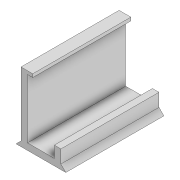
# Autodesk Inventor part: WagoHolder
Saved by Autodesk Inventor 2021 (Build 250183000, 183)
## iProperties
Created: 2021-07-30
Part Number: WagoHolder
Material: Generisch
Document SubType Name: Modeling
Designer: Rama
Density: 1 g/cm^3
Appearance: Vorgabe
Author: Rama
Autodesk Inventor part; units mm, degrees
ref_plane "YZ Plane" through (0, 0, 0) normal (1, 0, 0) x (0, 1, 0)
ref_plane "XZ Plane" through (0, 0, 0) normal (0, 1, 0) x (-1, 0, 0)
ref_plane "XY Plane" through (0, 0, 0) normal (0, 0, 1) x (1, 0, 0)
sketch "Skizze1" plane through (0, 0, 0) normal (0, 1, 0) x (-1, 0, 0)
  line L0 (4.1, 15) -> (-4.1, 15)
  line L1 (-4.1, 15) -> (-4.1, -15)
  line L2 (-4.1, -15) -> (4.1, -15)
  line L3 (4.1, -15) -> (4.1, 15)
  line L4 (4.1, 15) -> (-4.1, -15) construction
  line L5 (-4.1, 15) -> (4.1, -15) construction
  line L6 (6.1, 17) -> (-6.1, 17)
  line L7 (-6.1, 17) -> (-6.1, -17)
  line L8 (-6.1, -17) -> (6.1, -17)
  line L9 (6.1, -17) -> (6.1, 17)
  line L10 (6.1, 17) -> (-6.1, -17) construction
  line L11 (-6.1, 17) -> (6.1, -17) construction
  point P0 (0, 0)
  dimension "d0" = 8.2
  dimension "d1" = 30
  dimension "d2" = 12.2
  dimension "d3" = 34
  constraints: 24 end point, 4 midpoint, 4 parallel, 2 horizontal, 2 perpendicular
  measures "d0" distance of L2.end L1.end
  measures "d1" distance of L1.end L0.end
  measures "d2" distance of L8.end L7.end
  measures "d3" distance of L7.end L6.end
extrude "Extrusion1" add sketch "Skizze1" along normal blind 18.1
sketch "Skizze2" plane through (0, 0, 0) normal (0, -1, 0) x (1, 0, 0)
  line L0 (6.1, 17) -> (6.1, -17) projected
  line L1 (-6.1, 17) -> (6.1, 17) projected
  line L2 (-6.1, -17) -> (-6.1, 17) projected
  line L3 (6.1, -17) -> (-6.1, -17) projected
  line L4 (-4.1, 15) -> (-4.1, -15) projected
  line L5 (4.1, 15) -> (-4.1, 15) projected
  line L6 (4.1, -15) -> (4.1, 15) projected
  line L7 (-4.1, -15) -> (4.1, -15) projected
  point P0 (0, 0)
extrude "Extrusion2" add sketch "Skizze2" along normal blind 2 contours L0 L3 L2 L1 | L5 L6 L7 L4
sketch "Skizze3" plane through (6.1, 18.1, 17) normal (1, 0, 0) x (0, 0, -1)
  line L0 (2, -18.1) -> (32, -18.1) projected
  line L1 (32, -18.1) -> (32, 0) projected
  line L2 (2, 0) -> (32, 0) projected
  line L3 (2, -18.1) -> (2, 0) projected
  line L4 (32, -18.1) -> (32, 0) projected
  line L5 (2, -18.1) -> (32, -18.1)
  line L6 (32, -18.1) -> (32, -14.6)
  line L7 (32, -14.6) -> (2, -14.6)
  line L8 (2, -14.6) -> (2, -18.1)
  point P0 (17, -18.1)
  point P1 (2, -14.6)
  dimension "d8" = 3.5
  constraints: 8 end point, 2 parallel, 1 horizontal, 1 perpendicular, 1 point on line
  measures "d8" distance of L6.end L5.end
extrude "Extrusion3" cut sketch "Skizze3" against normal up to surface (2 mm away) contours L3 L2 L1 L7
sketch "Skizze4" plane through (0, 18.1, 0) normal (0, 1, 0) x (1, 0, 0)
  line L0 (-4.1, -15) -> (-4.1, 15) projected
  line L1 (4.1, -15) -> (-4.1, -15) projected
  line L2 (-4.1, 15) -> (-3.5, 15)
  line L3 (-3.5, 15) -> (-3.5, -15)
  line L4 (-3.5, -15) -> (-4.1, -15)
  line L5 (-4.1, -15) -> (-4.1, 15)
  line L6 (-3.5, 15) -> (-2.9, 15)
  line L7 (-2.9, 15) -> (-2.9, -15)
  line L8 (-2.9, -15) -> (-3.5, -15)
  line L9 (-3.5, -15) -> (-3.5, 15)
  line L10 (-6.1, 17) -> (6.1, 17) projected
  line L11 (-6.1, -17) -> (6.1, -17) projected
  line L12 (-6.1, 17) -> (-2.9, 17)
  line L13 (-2.9, 17) -> (-2.9, -17)
  line L14 (-2.9, -17) -> (-6.1, -17)
  line L15 (-6.1, -17) -> (-6.1, 17)
  point P0 (0, 0)
  dimension "d11" = 0.6
  dimension "d12" = 0.6
  constraints: 24 end point, 6 parallel, 3 horizontal, 3 perpendicular, 3 point on line
  measures "d11" distance of L3.end L4.end
  measures "d12" distance of L7.end L8.end
extrude "Extrusion4" add sketch "Skizze4" along normal blind 1
sketch "Skizze6" plane through (-4.1, 0, -15) normal (0, 0, 1) x (1, 0, 0)
  line L0 (10.2, -2) -> (10.2, 18.1) projected
  line L1 (0, 0) -> (0, 18.1) projected
  line L2 (10.2, 18.1) -> (0, 18.1)
  line L3 (0, 18.1) -> (0, 3.5)
  line L4 (0, 3.5) -> (10.2, 3.5)
  line L5 (10.2, 3.5) -> (10.2, 18.1)
  point P0 (4.1, 0)
  dimension "d30" = 14.6
  constraints: 8 end point, 2 parallel, 1 horizontal, 1 perpendicular, 1 point on line
  measures "d30" distance of L3.end L2.end
extrude "Extrusion6" cut sketch "Skizze6" against normal through all
mirror "Spiegeln1" about plane through (0, 0, 0) normal (0, 0, 1) of "Extrusion6"
sketch "Skizze7" plane through (-4.1, 0, -15) normal (0, 0, 1) x (1, 0, 0)
  line L0 (8.2, 3.5) -> (0, 3.5) projected
  line L1 (0, 0) -> (0, 3.5) projected
  line L2 (0, 0) -> (8.2, 0) projected
  line L3 (8.2, 0) -> (8.2, 3.5) projected
  point P0 (4.1, 0)
extrude "Extrusion7" cut sketch "Skizze7" along normal through all both and the other way through all
sketch "Skizze8" plane through (6.1, -2, -17) normal (0, 0, -1) x (-1, 0, 0)
  line L0 (2, 2) -> (2, 5.5) projected
  line L1 (2, 5.5) -> (0, 5.5) projected
  line L2 (0, 0) -> (0, 5.5) projected
  line L3 (12.2, 0) -> (0, 0) projected
  line L4 (12.2, 0) -> (12.2, 21.1) projected
  line L5 (9, 21.1) -> (12.2, 21.1) projected
  line L6 (9, 20.1) -> (9, 21.1) projected
  line L7 (9, 20.1) -> (10.2, 20.1) projected
  line L8 (10.2, 20.1) -> (10.2, 2) projected
  line L9 (10.2, 2) -> (2, 2) projected
  point P0 (6.1, 2)
extrude "Extrusion8" cut sketch "Skizze8" against normal blind 2
mirror "Spiegeln2" about plane through (0, 0, 0) normal (0, 0, 1) of "Extrusion8"
sketch "Skizze10" plane through (-6.1, -2, 15) normal (0, 0, 1) x (1, 0, 0)
  line L0 (12.2, 0) -> (0, 0) projected
  line L1 (0, 0) -> (-1.5, 0)
  line L2 (-1.5, 0) -> (-1.5, 1.5)
  line L3 (-1.5, 1.5) -> (0, 1.5)
  line L4 (0, 1.5) -> (0, 0)
  line L5 (12.2, 0) -> (13.7, 0)
  line L6 (13.7, 0) -> (13.7, 1.5)
  line L7 (13.7, 1.5) -> (12.2, 1.5)
  line L8 (12.2, 1.5) -> (12.2, 0)
  line L9 (0, 1.5) -> (-1.5, 0)
  line L10 (12.2, 1.5) -> (13.7, 0)
  point P0 (6.1, 2)
  dimension "d44" = 1.5
  dimension "d45" = 1.5
  dimension "d46" = 1.5
  dimension "d47" = 1.5
  constraints: 20 end point, 4 parallel, 2 horizontal, 2 perpendicular
  measures "d44" distance of L2.end L3.end
  measures "d45" distance of L1.end L2.end
  measures "d46" distance of L7.end L6.end
  measures "d47" distance of L6.end L5.end
extrude "Extrusion10" add sketch "Skizze10" against normal up to surface (30 mm away) contours L1 L9 L4 | L8 L10 L5
sketch "Skizze11" plane through (-2.9, 18.1, -15) normal (1, 0, 0) x (0, 0, -1)
  line L0 (-30, 1) -> (-30, 0) projected
  line L1 (0, 0) -> (-30, 0) projected
  line L2 (0, 0) -> (0, 1) projected
  line L3 (-30, 1) -> (0, 1) projected
  point P0 (-15, -18.1)
extrude "Extrusion11" add sketch "Skizze11" along normal blind 0.4
